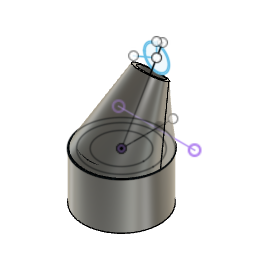
tobera (Autodesk Fusion 360 design; units mm, degrees)
Autodesk Fusion 360 part; units mm, degrees
sketch "Boceto1" plane through (0, 0, 0) normal (0, 0, 1) x (1, 0, 0)
  circle A0 centre (0, 0) radius 13.6
  circle A1 centre (0, 0) radius 9.5
  circle A2 centre (0, 0) radius 16.335
  dimension "d1" = 27.2
  dimension "d2" = 19
  dimension "d3" = 32.67
  constraint coincident A0.centre A1.centre
  constraint concentric A0 A1
  measures "d1" diameter of A0
  measures "d2" diameter of A1
  measures "d3" diameter of A2
sketch "Boceto2" plane through (0, 0, 0) normal (1, 0, 0) x (0, 1, 0)
  line L0 (0, 0) -> (0, 0.01)
  line L1 (0, 0.01) -> (17.6565, 30.592)
  line L2 (0, 0.01) -> (22.1326, 0.01) construction
  line L3 (0, 0) -> (16.3, 0)
  line L4 (15.11, 26.1813) -> (5.1943, 31.9061)
  line L5 (15.11, 26.1813) -> (15.11, 32.2745)
  dimension "d8" = 0.01
  dimension "d9" = 60
  dimension "d10" = 16.3
  constraint coincident L0.start L3.start
  constraint vertical L0
  constraint horizontal L2
  constraint perpendicular L0 L3
  constraint coincident L1 L4.start
  constraint perpendicular L1 L4
  constraint vertical L5
  measures "d8" distance of L0.start L0.end
  measures "d9" angle of L1 L2
  measures "d10" distance of L0.start L3.end
ref_plane "PlanoDeObra2" through (0, 15.11, 29.2279) normal (0, -1, 0) x (0, 0, 1)
sketch "Boceto3" plane through (0, 15.11, 0) normal (0, -1, 0) x (-1, 0, 0)
  circle A0 centre (-0.0084, -26.213) radius 5
  circle A1 centre (-0.0084, -26.213) radius 5.5
  line L0 (-16.335, 0) -> (16.335, 0)
  dimension "d15" = 10
  dimension "d16" = 11
  dimension "d19" = 26.213
  constraint concentric A0 A1
  measures "d15" diameter of A0
  measures "d16" diameter of A1
  measures "d19" distance of A0.centre L0
extrude "Extruir3" add sketch "Boceto1" against normal blind 5 contours A0 makes body 1
loft "Solevación1" add profiles "Boceto1", "Boceto3" section 1 contours A2 section 2 separate body makes body 2 in component "Component"
loft "Solevación3" cut profiles "Boceto1", "Boceto3" section 1 contours A1 section 2 contours A0 bodies 2 in component "Component"
extrude "Extruir4" add sketch "Boceto1" against normal blind 20 contours A2 bodies 1
ref_plane "PlanoDeObra4" through (0, 10.1522, 29.0437) normal (0, 0.5, 0.866025) x (0, -0.866025, 0.5)
ref_plane "PlanoDeObra5" through (0, 7.6522, 24.7136) normal (0, 0.5, 0.866025) x (0, -0.866025, 0.5)
sketch "Boceto5" plane through (0, 12.6143, 21.8487) normal (0, 0.5, 0.866025) x (0, -0.866025, 0.5)
  line L0 (14.7139, -12.2155) -> (-15.8463, -12.2155)
  line L1 (-15.8463, -12.2155) -> (-15.8463, 16.6589)
  line L2 (-15.8463, 16.6589) -> (14.7139, 16.6589)
  line L3 (14.7139, 16.6589) -> (14.7139, -12.2155)
  constraint horizontal L0
  constraint vertical L1
  constraint horizontal L2
  constraint vertical L3
extrude "Extruir1" cut sketch "Boceto5" along normal blind 25 bodies 2 in component "Component"
extrude "Extruir5" add sketch "Boceto1" along normal blind 2 separate body contours A0 makes body 3
component "Component" placed x (1, 0, 0) y (0, 1, 0) z (0, 0, 1) at (0, 0, 0)
